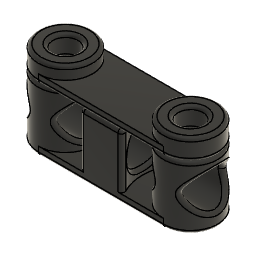
Coupler_Extender (Autodesk Fusion 360 design; units mm, degrees)
Autodesk Fusion 360 part; units mm, degrees
sketch "Sketch1" plane through (0, 0, 0) normal (0, 0, 1) x (1, 0, 0)
  circle A0 centre (-7.5, 0) radius 3.25
  circle A1 centre (7.5, 0) radius 3.25
  line L0 (0, 0) -> (7.5, 0)
  line L1 (0, 0) -> (-7.5, 0)
  line L2 (7.5, -3.25) -> (-7.5, -3.25)
  line L3 (-7.5, -3.25) -> (-7.5, 3.25)
  line L4 (-7.5, 3.25) -> (7.5, 3.25)
  line L5 (7.5, 3.25) -> (7.5, -3.25)
  line L6 (7.5, -3.25) -> (-7.5, 3.25) construction
  line L7 (-7.5, -3.25) -> (7.5, 3.25) construction
  line L8 (5.5, -3.25) -> (-5.5, -3.25)
  line L9 (-5.5, -3.25) -> (-5.5, 3.25)
  line L10 (-5.5, 3.25) -> (5.5, 3.25)
  line L11 (5.5, 3.25) -> (5.5, -3.25)
  line L12 (5.5, -3.25) -> (-5.5, 3.25) construction
  line L13 (-5.5, -3.25) -> (5.5, 3.25) construction
  circle A2 centre (7.5, 0) radius 5.75
  circle A3 centre (-7.5, 0) radius 5.75
  dimension "d1" = 6.5
  dimension "d2" = 6.5
  dimension "d3" = 15
  dimension "d4" = 7.5
  dimension "d5" = 15
  dimension "d6" = 6.5
  dimension "d11" = 11
  dimension "d12" = 6.5
  dimension "d15" = 11.5
  dimension "d16" = 11.5
  constraint coincident L0.start L1.start
  constraint coincident A1.centre L0.end
  constraint horizontal L0
  constraint coincident A0.centre L1.end
  constraint parallel L0 L1
  constraint horizontal L2
  constraint perpendicular L2 L3
  constraint parallel L2 L4
  constraint parallel L3 L5
  constraint coincident L6 L0.start
  constraint coincident L7 L0.start
  constraint horizontal L8
  constraint perpendicular L8 L9
  constraint parallel L8 L10
  constraint parallel L9 L11
  constraint coincident L12 L0.start
  constraint coincident L13 L0.start
  constraint concentric A1 A2
  constraint concentric A0 A3
  measures "d1" diameter of A0
  measures "d2" diameter of A1
  measures "d3" distance of A0.centre A1.centre
  measures "d4" distance of L0.start A0.centre
  measures "d5" distance of L3.end L4.end
  measures "d6" distance of L2.end L3.end
  measures "d11" distance of L9.end L10.end
  measures "d12" distance of L8.end L9.end
  measures "d15" diameter of A2
  measures "d16" diameter of A3
extrude "Extrude1" add sketch "Sketch1" along normal blind 7.5 contours A0 L3 | A0 L1 L3 L9 | A0 L1 L3 L9 | A0 L1 L9 | A0 L1 L9 | A1 L0 L5 L11 | A1 L5 | A1 L0 L11 | A1 L0 L11 | A1 L0 L5 L11 makes body 1 at (-4.2661, -0.3236, 2.5) makes body 2 at (10.7339, -0.3236, 2.5)
extrude "Extrude2" add sketch "Sketch1" along normal blind 1 contours A0 L4 L9 | A0 L2 L9 | A0 L1 L4 L9 L10 A3 | A0 L1 L2 L8 L9 A3 | L0 L1 L4 L10 A2 A3 | L0 L1 L2 L8 A2 A3 | A1 L0 L4 L10 L11 A2 | A1 L0 L2 L8 L11 A2 | A1 L4 L11 | A1 L2 L11 bodies 1 2
extrude "Extrude3" add sketch "Sketch1" along normal blind 7.5 contours L0 L1 L4 L10 A2 A3 | L0 L1 L2 L8 A2 A3 bodies 1
sketch "Sketch2" plane through (0, 0, 7.5) normal (0, 0, 1) x (-1, 0, 0)
  circle A0 centre (7.5, 0) radius 3.25
  circle A1 centre (-7.5, 0) radius 3.25
  line L0 (7.5, -3.25) -> (-7.5, -3.25)
  line L1 (7.5, 3.25) -> (-7.5, 3.25)
  constraint coincident A0 L0.start
  constraint coincident A1 L0.end
  constraint tangent A1 L0
  constraint horizontal L0
  constraint coincident A0 L1.start
  constraint coincident A1 L1.end
  constraint tangent A1 L1
  constraint parallel L0 L1
extrude "Extrude4" add sketch "Sketch2" along normal blind 1 separate body makes body 3
ref_plane "WorkPlane1" through (-15, 0, 0) normal (1, 0, 0) x (0, 1, 0)
sketch "Sketch3" plane through (-15, 0, 0) normal (1, 0, 0) x (0, 1, 0)
  circle A0 centre (0, 4) radius 2.25
  line L0 (3.25, 0) -> (-3.25, 0)
  line L1 (-3.25, 1) -> (-3.25, 7.5)
  dimension "d20" = 4.5
  dimension "d21" = 4
  dimension "d22" = 3.25
  measures "d20" diameter of A0
  measures "d21" distance of A0.centre L0
  measures "d22" distance of A0.centre L1
extrude "Extrude5" cut sketch "Sketch3" along normal blind 32 bodies 1
fillet "Fillet1" radius 0.4 10 edges at (2.7566, -3.25, 4.25) (2.7566, 3.25, 4.25) (-2.7566, 3.25, 4.25) (-2.7566, -3.25, 4.25) (-2.2085, -2.25, 4) (2.2085, -2.25, 4) (5.1548, -2.25, 4) (9.8452, -2.25, 4) (-5.1548, -2.25, 4) (-9.8452, -2.25, 4) 4 faces at (-6.7001, 0.3017, 7.5) (0.5876, 0.8903, 7.5) (8.5712, -0.7786, 7.5) (2.5, 1.0833, 0) on bodies 1
sketch "Sketch4" plane through (0, 0, 8.5) normal (0, 0, 1) x (-1, 0, 0)
  arc A0 (7.5, -3.25) -> (7.5, 3.25) centre (7.5, 0) ccw
  line L0 (7.5, 3.25) -> (-7.5, 3.25)
  arc A1 (-7.5, 3.25) -> (-7.5, -3.25) centre (-7.5, 0) ccw
  line L1 (-7.5, -3.25) -> (7.5, -3.25)
  circle A2 centre (7.5, 0) radius 3.25
  circle A3 centre (-7.5, 0) radius 3.25
  dimension "d29" = 6.5
  dimension "d30" = 6.5
  constraint concentric A0 A2
  constraint concentric A1 A3
  measures "d29" diameter of A2
  measures "d30" diameter of A3
extrude "Extrude6" add sketch "Sketch4" along normal blind 1.5 contours A0 A2 | A1 A3 bodies 3
sketch "Sketch5" plane through (0, 0, 10) normal (0, 0, 1) x (-1, 0, 0)
  circle A0 centre (7.5, 0) radius 3.25
  circle A1 centre (7.5, 0) radius 1.5
  circle A2 centre (-7.5, 0) radius 3.25
  circle A3 centre (-7.5, 0) radius 1.5
  dimension "d33" = 3
  dimension "d34" = 3
  constraint concentric A0 A1
  constraint concentric A2 A3
  measures "d33" diameter of A1
  measures "d34" diameter of A3
extrude "Extrude7" cut sketch "Sketch5" against normal blind 3.5 contours A1 | A3 bodies 3
sketch "Sketch6" plane through (0, 0, 7.5) normal (0, 0, 1) x (-1, 0, 0)
  circle A0 centre (7.5, 0) radius 2.85
  circle A1 centre (-7.5, 0) radius 2.85
  circle A2 centre (7.5, 0) radius 1.25
  circle A3 centre (-7.5, 0) radius 1.25
  dimension "d37" = 2.5
  dimension "d38" = 2.5
  constraint concentric A0 A2
  constraint concentric A1 A3
  measures "d37" diameter of A2
  measures "d38" diameter of A3
extrude "Extrude8" cut sketch "Sketch6" against normal blind 3 contours A2 | A3 bodies 1
fillet "Fillet3" radius 0.4 12 edges at (-6.3346, -0.452, 7.5) (8.6654, -0.452, 7.5) (-4.4699, 1.1753, 10) (10.5301, 1.1753, 10) (8.8985, -0.5424, 10) (-6.1015, -0.5424, 10) (0, 3.25, 7.5) (-10.75, 0, 7.5) (0, -3.25, 7.5) (10.75, 0, 7.5) (-6.1015, 0.5424, 7.5) (8.8985, 0.5424, 7.5) on bodies 1 3
equation "d4 = d3 / 2"
equation "d5 = d3"
equation "d6 = d1"
equation "d12 = d1"
equation "d16 = d15"
named bodies: "Extender", "Cap"
